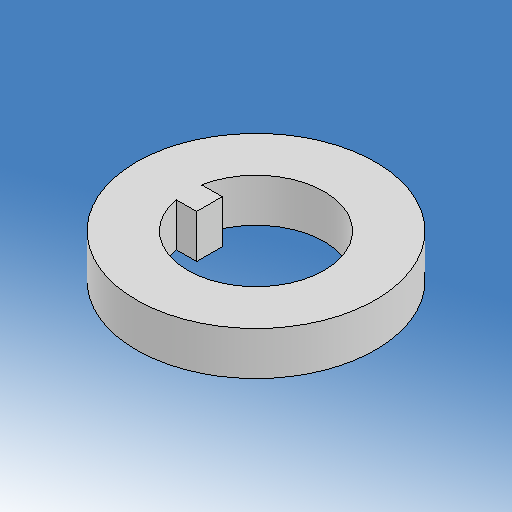
# Autodesk Inventor part: 8mKeyyedShaftSpacer_BevelToSpurShaft
Saved by Autodesk Inventor 2025 (Build 290162000, 162)
## iProperties
Created: 2024-06-12
Part Number: 8mKeyyedShaftSpacer_BevelToSpurShaft
Material: Generic
Document SubType Name: Modeling
Designer: seene
Density: 1 g/cm^3
Appearance: Default
Author: seene
Autodesk Inventor part; units mm, degrees
ref_plane "YZ Plane" through (0, 0, 0) normal (1, 0, 0) x (0, 1, 0)
ref_plane "XZ Plane" through (0, 0, 0) normal (0, 1, 0) x (-1, 0, 0)
ref_plane "XY Plane" through (0, 0, 0) normal (0, 0, 1) x (1, 0, 0)
sketch "Sketch1" plane through (0, 0, 0) normal (0, 1, 0) x (-1, 0, 0)
  circle A0 centre (0, 0) radius 4
  circle A1 centre (0, 0) radius 7
  line L0 (3.9291, 0.75) -> (2.7291, 0.75)
  line L1 (2.7291, 0.75) -> (2.7291, -0.75)
  line L2 (2.7291, -0.75) -> (3.9291, -0.75)
  line L3 (3.9291, -0.75) -> (3.9291, 0.75)
  line L4 (3.9291, 0) -> (2.7291, 0) construction
  line L5 (0, 0) -> (-4, 0) construction
  dimension "d0" = 8
  dimension "d1" = 3
  dimension "d2" = 1.2
  dimension "d3" = 1.5
  constraints: 12 end point, 2 centre point, 2 horizontal, 2 midpoint, 2 parallel, 2 point on circle, 1 coincident, 1 collinear, 1 perpendicular
  measures "d0" diameter of A0
  measures "d1" radial gap between concentric circles of A0 A1
  measures "d2" distance of L1.end L2.end
  measures "d3" distance of L0.end L1.end
extrude "Extrusion1" add sketch "Sketch1" along normal blind 2.54 contours A0 L3 | L3 L2 L1 L0 | A1
body "Solid1"
